DHEClockingcap (Autodesk Fusion 360 design; units mm, degrees)
Autodesk Fusion 360 part; units mm, degrees
sketch "Sketch1" plane through (0, 0, 0) normal (0, 0, 1) x (1, 0, 0)
  circle A0 centre (0, 0) radius 60
  circle A1 centre (0, 0) radius 5
  dimension "d10" = 10
  constraint coincident A0.centre A1.centre
  constraint concentric A0 A1
  measures "d10" diameter of A1
extrude "Extrude1" add sketch "Sketch1" along normal blind 5
thread "Thread1" "BSP Pipe Threads G 2-11" major diameter 59.434 minor diameter 56.656 pitch 2.3091 angle 55 resizes the face on face at (59.9254, -2.9908, 3.3333)
sketch "Sketch2" plane through (0, 0, 0) normal (0, 0, -1) x (1, 0, 0)
  circle A0 centre (0, 0) radius 29.717
  line L0 (25, 7.5) -> (28, 7.5)
  line L1 (28, 7.5) -> (28, -7.5)
  line L2 (28, -7.5) -> (25, -7.5)
  line L3 (25, -7.5) -> (25, 7.5)
  circle A1 centre (0, 0) radius 5
  point P0 (25, 0)
  dimension "d3" = 3
  dimension "d4" = 15
  dimension "d5" = 25
  constraint horizontal L0
  constraint vertical L1
  constraint horizontal L2
  constraint vertical L3
  constraint midpoint L3 P0
  constraint horizontal A0.centre P0
  measures "d3" distance of L1 L3
  measures "d4" distance of L0 L2
  measures "d5" distance of A0.centre L3
extrude "Extrude2" add sketch "Sketch2" along normal blind 15 contours L0 L1 L2 L3
sketch "Sketch3" plane through (28, 0, 0) normal (1, 0, 0) x (0, 1, 0)
  line L0 (7.5, 0) -> (-7.5, 0)
  line L1 (-7.5, 0) -> (-7.5, -15)
  line L2 (-7.5, -15) -> (7.5, -15)
  line L3 (7.5, -15) -> (7.5, 0)
  circle A0 centre (0, -7.5) radius 5
  circle A1 centre (0, -7.5) radius 7.5
  dimension "d8" = 10
  constraint concentric A0 A1
  constraint tangent L1 A1
  constraint tangent L3 A1
  constraint tangent L2 A1
  measures "d8" diameter of A0
extrude "Extrude3" cut sketch "Sketch3" against normal through all contours L2 L3 A1 | L1 L2 A1 | A0
